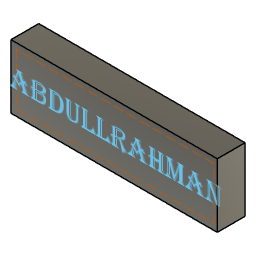
Untitled v1 (Autodesk Fusion 360 design; units mm, degrees)
Autodesk Fusion 360 part; units mm, degrees
sketch "Sketch1" plane through (0, 0, 0) normal (0, 1, 0) x (1, 0, 0)
  line L0 (0, 0) -> (74.1987, 0)
  line L1 (74.1987, 0) -> (74.1987, -22.9176)
  line L2 (74.1987, -22.9176) -> (0, -22.9176)
  line L3 (0, -22.9176) -> (0, 0)
  constraint horizontal L0
  constraint vertical L1
  constraint horizontal L2
  constraint vertical L3
  constraint coincident L0.start L3.end
extrude "Extrude1" add sketch "Sketch1" along normal blind 10
sketch "Sketch2" plane through (0, 0, 0) normal (0, 1, 0) x (1, 0, 0)
  line L0 (2.0422, -2.2691) -> (73.0641, -2.2691) construction
  line L1 (73.0641, -2.2691) -> (73.0641, -20.8755) construction
  line L2 (73.0641, -20.8755) -> (2.0422, -20.8755) construction
  line L3 (2.0422, -20.8755) -> (2.0422, -2.2691) construction
  dimension "d3" = 6.5
